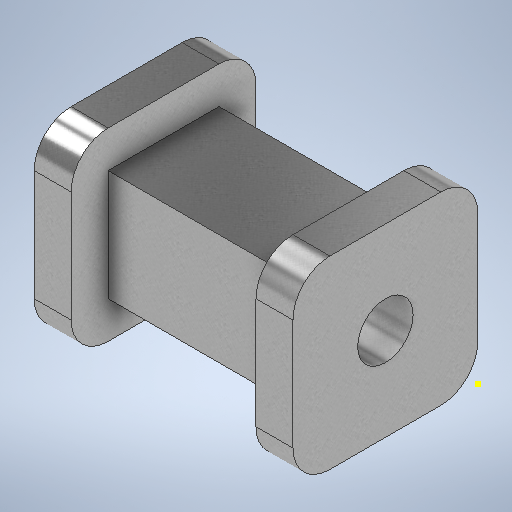
# Autodesk Inventor part: Contenedor
Saved by Autodesk Inventor 2025.1 (Build 291241000, 241)
## iProperties
Created: 2025-02-26
Part Number: Contenedor
Material: Generic
Document SubType Name: Modeling
Designer: yovan
Density: 1 g/cm^3
Appearance: Default
Author: yovan
Autodesk Inventor part; units mm, degrees
ref_plane "YZ Plane" through (0, 0, 0) normal (1, 0, 0) x (0, 1, 0)
ref_plane "XZ Plane" through (0, 0, 0) normal (0, 1, 0) x (-1, 0, 0)
ref_plane "XY Plane" through (0, 0, 0) normal (0, 0, 1) x (1, 0, 0)
sketch "Sketch1" plane through (0, 0, 0) normal (1, 0, 0) x (0, 1, 0)
  line L0 (0, 0) -> (50, 0)
  line L1 (50, 0) -> (50, 50)
  line L2 (50, 50) -> (0, 50)
  line L3 (0, 50) -> (0, 0)
  circle A0 centre (25, 25) radius 7.5
  dimension "d0" = 50
  dimension "d1" = 50
  dimension "d2" = 15
  constraints: 8 end point, 2 parallel, 1 centre point, 1 horizontal, 1 perpendicular
  measures "d0" distance of L2.end L1.end
  measures "d1" distance of L1.end L0.end
  measures "d2" diameter of A0
extrude "Extrusion1" add sketch "Sketch1" along normal blind 60
extrude "Extrusion7" add sketch "Sketch1" against normal blind 10 contours L3 L2 L1 L0 | A0
sketch "Sketch6" plane through (60, 0, 50) normal (0, 0, 1) x (1, 0, 0)
  line L0 (0, 50) -> (-70, 50) projected
  line L1 (-70, 0) -> (0, 0) projected
  line L2 (-60, 50) -> (-10, 50)
  line L3 (-10, 50) -> (-10, 0)
  line L4 (-10, 0) -> (-60, 0)
  line L5 (-60, 0) -> (-60, 50)
  line L6 (-60, 50) -> (-10, 50)
  line L7 (-10, 50) -> (-10, 40)
  line L8 (-10, 40) -> (-60, 40)
  line L9 (-60, 40) -> (-60, 50)
  line L10 (-10, 0) -> (-60, 0)
  line L11 (-60, 0) -> (-60, 10)
  line L12 (-60, 10) -> (-10, 10)
  line L13 (-10, 10) -> (-10, 0)
  line L14 (-60, 50) -> (-10, 50)
  line L15 (-10, 50) -> (-10, 0)
  line L16 (-10, 0) -> (-60, 0)
  line L17 (-60, 0) -> (-60, 50)
  point P0 (-10, 10)
  dimension "d33" = 50
  dimension "d34" = 10
  dimension "d35" = 10
  constraints: 32 end point, 8 parallel, 4 horizontal, 4 perpendicular, 4 point on line
  measures "d33" distance of L3.end L4.end
  measures "d34" distance of L6.end L7.end
  measures "d35" distance of L10.end L11.end
extrude "Extrusion8" cut sketch "Sketch6" against normal blind 100 contours L3 L8 L5 L0 | L3 L1 L5 L12
extrude "Extrusion9" cut sketch "Sketch6" against normal blind 10 contours L3 L12 L5 L8
sketch "Sketch7" plane through (60, 0, 0) normal (0, 0, -1) x (-1, 0, 0)
  line L0 (60, 10) -> (60, 40) projected
  line L1 (10, 0) -> (10, 10) projected
  line L2 (60, 40) -> (10, 40)
  line L3 (10, 40) -> (10, 10)
  line L4 (10, 10) -> (60, 10)
  line L5 (60, 10) -> (60, 40)
  point P0 (60, 0)
  constraints: 8 end point, 2 parallel, 1 horizontal, 1 perpendicular
extrude "Extrusion10" cut sketch "Sketch7" against normal blind 10
fillet "Fillet4" radius 10 8 edges at (55, 50, 50) (-5, 50, 50) (-5, 50, 0) (55, 0, 50) (55, 50, 0) (-5, 0, 50) (55, 0, 0) (-5, 0, 0)
sketch "Sketch8" plane through (60, 0, 0) normal (1, 0, 0) x (0, 0, -1)
  point P0 (0, 0)
body "Solid1"
